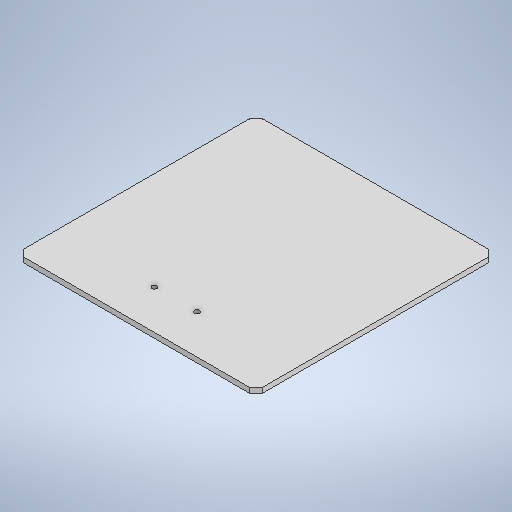
# Autodesk Inventor part: table
Saved by Autodesk Inventor 2027 (Build 310192060, 192F)
## iProperties
Created: 2026-05-28
Part Number: table
Material: Generic
Document SubType Name: Modeling
Designer: savas
Density: 1 g/cm^3
Appearance: Default
Author: savas
Autodesk Inventor part; units mm, degrees
ref_plane "YZ Plane" through (0, 0, 0) normal (1, 0, 0) x (0, 1, 0)
ref_plane "XZ Plane" through (0, 0, 0) normal (0, 1, 0) x (-1, 0, 0)
ref_plane "XY Plane" through (0, 0, 0) normal (0, 0, 1) x (1, 0, 0)
sketch "Sketch1" plane through (0, 0, 0) normal (0, 1, 0) x (-1, 0, 0)
  line L0 (0, 0) -> (140, 0)
  line L1 (140, 0) -> (140, -140)
  line L2 (140, -140) -> (0, -140)
  line L3 (0, -140) -> (0, 0)
  circle A0 centre (82.5, -23) radius 1.5
  circle A1 centre (57.5, -23) radius 1.5
  line L4 (82.5, -23) -> (57.5, -23) construction
  point P0 (70, -23)
  point P1 (70, 0)
  dimension "d0" = 140
  dimension "d1" = 140
  dimension "d2" = 3
  dimension "d3" = 23
  dimension "d4" = 25
  constraints: 10 end point, 2 centre point, 2 horizontal, 2 midpoint, 2 parallel, 1 equal radius, 1 horizontal alignment, 1 perpendicular, 1 vertical alignment
  measures "d0" distance of L1.end L2.end
  measures "d1" distance of L0.end L1.end
  measures "d2" diameter of A0
  measures "d3" distance from line of L4.start L0
  measures "d4" distance of L4.end L4.start
extrude "Extrusion1" add sketch "Sketch1" along normal blind 3
chamfer "Chamfer1" distance 4 angle 45 4 edges at (-140, 1.5, 0) (-140, 1.5, -140) (0, 1.5, -140) (0, 1.5, 0)
body "Solid1"
